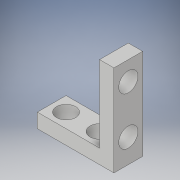
# Autodesk Inventor part: Servo Locks V3
Saved by Autodesk Inventor 2019 (Build 230136000, 136)
## iProperties
Created: 2018-11-14
Part Number: Servo Locks V3
Material: Generic
Document SubType Name: Modeling
Designer: Ashley
Density: 1 g/cm^3
Appearance: Default
Author: Ashley
Autodesk Inventor part; units mm, degrees
ref_plane "YZ Plane" through (0, 0, 0) normal (1, 0, 0) x (0, 1, 0)
ref_plane "XZ Plane" through (0, 0, 0) normal (0, 1, 0) x (-1, 0, 0)
ref_plane "XY Plane" through (0, 0, 0) normal (0, 0, 1) x (1, 0, 0)
sketch "Sketch1" plane through (0, 0, 0) normal (0, 1, 0) x (-1, 0, 0)
  line L0 (-9.5, -3) -> (6.5, -3)
  line L1 (6.5, -3) -> (6.5, 3)
  line L2 (6.5, 3) -> (-9.5, 3)
  line L3 (-9.5, 3) -> (-9.5, -3)
  circle A0 centre (3.5, 0) radius 2
  circle A1 centre (-3.5, 0) radius 2
  point P0 (0, 0)
  dimension "d0" = 4
  dimension "d3" = 3.5
  dimension "d4" = 4
  dimension "d5" = 3.5
  dimension "d6" = 7
  dimension "d7" = 6
  dimension "d8" = 3
  dimension "d9" = 3
  dimension "d10" = 3
  dimension "d11" = 6
  constraints: 8 end point, 2 centre point, 2 parallel, 1 horizontal, 1 perpendicular
  measures "d0" diameter of A0
  measures "d3" distance of point (0, 0) A0.centre
  measures "d4" diameter of A1
  measures "d5" distance of A1.centre point (0, 0)
  measures "d6" distance of A1.centre A0.centre
  measures "d7" distance of L2.end L0.start
  measures "d8" distance from line of L0 A1.centre
  measures "d9" distance from line of L2 A0.centre
  measures "d10" distance from line of A0.centre L1
  measures "d11" distance from line of A1.centre L3
extrude "Bottom Extrusion" add sketch "Sketch1" along normal blind 3
sketch "Sketch2" plane through (0, 3, 0) normal (0, 1, 0) x (1, 0, 0)
  line L0 (-6.5, -3) -> (9.5, -3) construction
  line L1 (9.5, -3) -> (9.5, 3) construction
  line L2 (9.5, 3) -> (6.5, 3)
  line L3 (6.5, 3) -> (6.5, -3)
  line L4 (6.5, -3) -> (9.5, -3)
  line L5 (9.5, -3) -> (9.5, 3)
  point P0 (0, 0)
  dimension "d14" = 3
  constraints: 8 end point, 2 parallel, 1 horizontal, 1 perpendicular, 1 point on line
  measures "d14" distance between parallel lines of L1 L3
extrude "Top Extrusion" add sketch "Sketch2" along normal blind 16
sketch "Sketch3" plane through (9.5, 0, 3) normal (1, 0, 0) x (0, 0, -1)
  line L0 (0, 19) -> (6, 19) construction
  circle A0 centre (3, 5) radius 2
  circle A1 centre (3, 15) radius 2
  point P0 (3, 0)
  dimension "d17" = 4
  dimension "d18" = 5
  dimension "d19" = 4
  dimension "d20" = 10
  dimension "d21" = 4
  constraints: 2 centre point
  measures "d17" diameter of A0
  measures "d18" distance of point (3, 0) A0.centre
  measures "d19" diameter of A1
  measures "d20" distance of A0.centre A1.centre
  measures "d21" distance from line of L0 A1.centre
extrude "Top Holes" cut sketch "Sketch3" against normal through all
body "Solid1"
